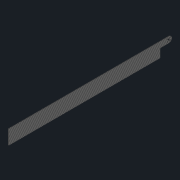
# Autodesk Inventor part: s_carbon_plate5
Saved by Autodesk Inventor 2022 (Build 260153000, 153)
## iProperties
Created: 2021-08-20
Part Number: s_carbon_plate5
Material: CFRP
Document SubType Name: Sheet Metal
Designer: yuta0
Density: 1.43 g/cm^3
Sheet Metal Rule: Default_mm
Appearance: カーボンファイバー
Author: yuta0
Autodesk Inventor part; units mm, degrees
ref_plane "YZ Plane" through (0, 0, 0) normal (1, 0, 0) x (0, 1, 0)
ref_plane "XZ Plane" through (0, 0, 0) normal (0, 1, 0) x (-1, 0, 0)
ref_plane "XY Plane" through (0, 0, 0) normal (0, 0, 1) x (1, 0, 0)
sketch "スケッチ1" plane through (0, 0, 0) normal (1, 0, 0) x (0, 1, 0)
  line L0 (-24.5, 275) -> (24.5, 275)
  line L1 (24.5, 275) -> (24.5, -275)
  line L2 (24.5, -275) -> (-24.5, -275)
  line L3 (-24.5, -275) -> (-24.5, 275)
  line L4 (-24.5, 275) -> (24.5, -275) construction
  line L5 (24.5, 275) -> (-24.5, -275) construction
  point P0 (0, 0)
  dimension "d0" = 49
  dimension "d1" = 550
  measures "d0" distance of L0.start L0.end
  measures "d1" distance of L0.end L1.end
extrude "プレート1" add sketch "スケッチ1" along normal mid plane 1
sketch "スケッチ3" plane through (0.5, 0, 0) normal (1, 0, 0) x (0, 0, -1)
  circle A0 centre (265, 14.5) radius 6
  line L0 (275, 24.5) -> (275, -24.5) projected
  line L1 (-275, 24.5) -> (275, 24.5) projected
  point P0 (0, 0)
  point P1 (269.2426, 18.7426)
  point P2 (260.7574, 18.7426)
  point P3 (260.7574, 10.2574)
  point P4 (269.2426, 10.2574)
  dimension "d13" = 12
  dimension "d14" = 10
  dimension "d15" = 10
  dimension "d18" = 360
  dimension "d30" = 0
  constraints: 8 other
  measures "d14" distance from line of L0 point (265, 14.5)
  measures "d15" distance from line of L1 point (265, 14.5)
  measures "d30" vertical distance of point (260.757, 18.743) point (269.243, 18.743)
hole "穴2" at (0.5, 18.7426, -269.2426) at (0.5, 18.7426, -260.7574) at (0.5, 10.2574, -260.7574) at (0.5, 10.2574, -269.2426) direction (-1, 0, 0) diameter 3.2 end through all clearance for "Socket Head Cap Screw" size "M3" standard "Ansi Metric M Profile"
sketch "スケッチ4" plane through (0.5, 0, 0) normal (1, 0, 0) x (0, 0, -1)
  circle A0 centre (265, 14.5) radius 3.05
  point P0 (0, 0)
  dimension "d27" = 6.1
  constraints: 1 centre point, 1 coincident
  measures "d27" diameter of A0
extrude "押し出し1" cut sketch "スケッチ4" against normal blind 10
sketch "スケッチ5" plane through (0.5, 0, 0) normal (1, 0, 0) x (0, 0, -1)
  line L0 (275, -24.5) -> (236, -24.5)
  line L1 (236, -24.5) -> (236, 4.5)
  line L2 (236, 4.5) -> (275, 4.5)
  line L3 (275, 4.5) -> (275, -24.5)
  line L4 (-275, 24.5) -> (216, 24.5)
  line L5 (216, 24.5) -> (216, 4.5)
  line L6 (216, 4.5) -> (-275, 4.5)
  line L7 (-275, 4.5) -> (-275, 24.5)
  line L8 (275, -24.5) -> (-275, -24.5) projected
  circle A0 centre (265, 14.5) radius 3.05 projected
  point P0 (0, 0)
  dimension "d35" = 29
  dimension "d36" = 20
  dimension "d40" = 29
  dimension "d41" = 10
  constraints: 16 end point, 4 parallel, 2 horizontal, 2 perpendicular
  measures "d35" distance between parallel lines of L8 L6
  measures "d36" distance between parallel lines of L1 L5
  measures "d40" distance from line of A0.centre L1
  measures "d41" distance from line of L2 A0.centre
extrude "押し出し2" cut sketch "スケッチ5" against normal blind 10 contours L0 L1 L2 L3
fillet "コーナーR2" radius 10 2 edges at (0, 24.5, -275) (0, 4.5, -275)
fillet "コーナーR3" radius 2 3 edges at (0, 4.5, -236) (0, -24.5, -236) (0, -24.5, 275)
equation "\"d15\" = d14"
equation "\"d25\" = Thickness"
equation "\"d2\" = Thickness"
equation "\"BendRadius\" = Thickness"
equation "\"BendReliefWidth\" = Thickness"
equation "\"BendReliefDepth\" = 0.5 * Thickness"
equation "\"CornerReliefSize\" = 4 * Thickness"
equation "\"MinimumRemnant\" = 2 * Thickness"
equation "\"TransitionRadius\" = BendRadius"
equation "\"JacobiRadiusSize\" = BendRadius"
equation "\"GapSize\" = Thickness"
equation "\"Thickness\" = 1"
